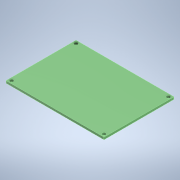
# Autodesk Inventor part: Plaquinha
Saved by Autodesk Inventor 2021 (Build 250183000, 183)
## iProperties
Created: 2022-02-21
Part Number: Plaquinha
Material: Generic
Document SubType Name: Modeling
Designer: Matheus
Density: 8.40429 g/cm^3
Appearance: Default
Mass: 46.8 g
Surface Area: 73.95 cm^2
Volume: 5.56858 cm^3
Author: Matheus
Autodesk Inventor part; units mm, degrees
ref_plane "YZ Plane" through (0, 0, 0) normal (1, 0, 0) x (0, 1, 0)
ref_plane "XZ Plane" through (0, 0, 0) normal (0, 1, 0) x (-1, 0, 0)
ref_plane "XY Plane" through (0, 0, 0) normal (0, 0, 1) x (1, 0, 0)
sketch "Sketch1" plane through (0, 0, 0) normal (0, 1, 0) x (-1, 0, 0)
  line L0 (-35, 25) -> (35, 25)
  line L1 (35, 25) -> (35, -25)
  line L2 (35, -25) -> (-35, -25)
  line L3 (-35, -25) -> (-35, 25)
  line L4 (-35, 25) -> (35, -25) construction
  line L5 (35, 25) -> (-35, -25) construction
  point P0 (0, 0)
  dimension "d0" = 70
  dimension "d1" = 50
  constraints: 12 end point, 2 midpoint, 2 parallel, 1 horizontal, 1 perpendicular
  measures "d0" distance of L1.end L2.end
  measures "d1" distance of L0.end L1.end
extrude "Extrusion1" add sketch "Sketch1" along normal blind 1.6
sketch "Sketch2" plane through (0, 1.6, 0) normal (0, 1, 0) x (1, 0, 0)
  line L0 (-49, 0) -> (49, 0) construction
  line L1 (0, 35) -> (0, -35) construction
  line L2 (-35, 25) -> (-35, -25) construction
  line L3 (-35, -25) -> (35, -25) construction
  point P0 (0, 0)
  point P1 (-33, -23)
  point P2 (33, -23)
  point P3 (-33, 23)
  point P4 (33, 23)
  dimension "d4" = 2
  dimension "d5" = 2
  constraints: 3 symmetric about line
  measures "d4" distance from line of L2 point (-33, -23)
  measures "d5" distance from line of L3 point (-33, -23)
hole "Hole1" at (-33, 1.6, 23) at (33, 1.6, 23) at (-33, 1.6, -23) at (33, 1.6, -23) direction (0, -1, 0) diameter 2.5 depth 1.6
body "Solid1"
